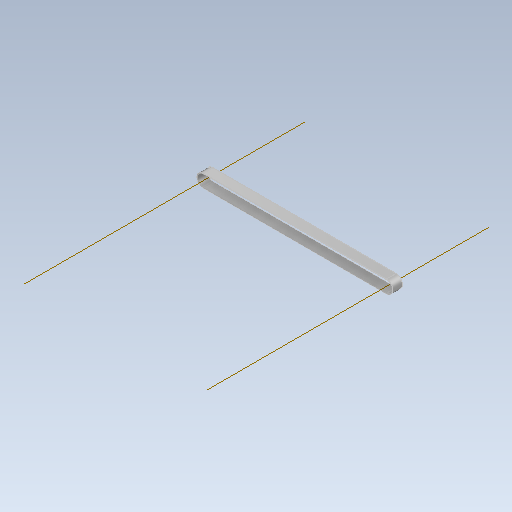
# Autodesk Inventor part: Correa síncrona
Saved by Autodesk Inventor 2021 (Build 250183000, 183)
## iProperties
Created: 2022-10-24
Part Number: Correa síncrona
Material: Rubber
Document SubType Name: Modeling
Designer: ivanm
Density: 1 g/cm^3
Appearance: Rubber - Black - Version 1.1
CustomPartVersion: 1
Author: ivanm
Autodesk Inventor part; units mm, degrees
sketch "Trayectoria de boceto" plane through (0, 0, 0) normal (0, 0, 1) x (1, 0, 0)
  arc A0 (-91.25, 6.3662) -> (-91.25, -6.3662) centre (-91.25, 0) ccw
  arc A1 (98.75, -6.3662) -> (98.75, 6.3662) centre (98.75, 0) ccw
  line L0 (98.75, -6.3662) -> (-91.25, -6.3662)
  line L1 (-91.25, 6.3662) -> (98.75, 6.3662)
  constraints: 4 end point, 4 point on circle, 2 centre point
ref_plane "Plano de sección transversal" through (-91.25, -6.3662, 0) normal (1, 0, 0) x (0, 0, 1)
ref_plane "Plano de trabajo2" through (-91.25, 0, 0) normal (-1, 0, 0) x (0, 0, 1)
ref_plane "Plano de trabajo3" through (98.75, 0, 0) normal (-0.9239, 0.3827, 0) x (0, 0, 1)
sketch "Sección transversal" plane through (-91.25, -6.3662, 0) normal (1, 0, 0) x (0, 0, 1)
  line L0 (-5, 0.3) -> (5, 0.3)
  line L1 (5, 0.3) -> (5, -0.3)
  line L2 (5, -0.3) -> (-5, -0.3)
  line L3 (-5, -0.3) -> (-5, 0.3)
  line L4 (-5, 0) -> (5, 0) construction
  point P0 (0, 0)
  point P1 (0, 0)
  dimension "d0" = 10
  dimension "d4" = 0.3
  dimension "d5" = 0.3
  constraints: 10 end point, 3 midpoint, 2 parallel, 1 coincident, 1 horizontal, 1 perpendicular, 1 other
  measures "d0" distance between parallel lines of L1 L3
  measures "d4" distance between parallel lines of L2 L4
  measures "d5" distance between parallel lines of L4 L0
sweep "Correa" add profiles "Sección transversal" path "Trayectoria de boceto"
equation "\"d0\" = da_B"
equation "\"d4\" = da_a"
equation "\"d5\" = da_a2"
equation "\"da_B\" = 10"
equation "\"da_pb\" = 2.5"
equation "\"da_a\" = 0.3"
equation "\"da_S\" = 1.5"
equation "\"da_Beta\" = 20deg"
equation "\"da_Ht\" = 0.7"
equation "\"da_H\" = 1.3"
equation "\"da_a2\" = 0.3"
body "Solid1"
